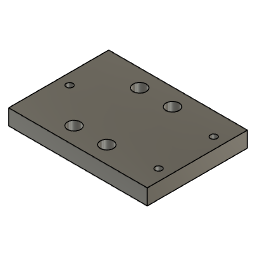
Fixation_camera v4 (Autodesk Fusion 360 design; units mm, degrees)
Autodesk Fusion 360 part; units mm, degrees
sketch "Esquisse1" plane through (0, 0, 0) normal (0, 0, 1) x (1, 0, 0)
  circle A0 centre (-12.5, 4.445) radius 2.5
  circle A1 centre (-12.5, -8.055) radius 2.5
  circle A2 centre (12.5, 4.445) radius 2.5
  circle A3 centre (-10.5, 22.15) radius 1.25
  line L0 (-14.5, -24.35) -> (-14.5, 24.35) construction
  line L1 (19.05, -25.4) -> (19.05, 25.4)
  line L2 (-19.05, -25.4) -> (-19.05, 25.4)
  circle A4 centre (12.5, -8.055) radius 2.5
  line L3 (-19.05, -25.4) -> (19.05, -25.4)
  line L4 (-19.05, 25.4) -> (-19.05, -25.4)
  line L5 (14.5, 24.35) -> (14.5, -24.35) construction
  line L6 (19.05, 25.4) -> (19.05, -25.4)
  line L7 (19.05, 25.4) -> (-19.05, 25.4)
  circle A5 centre (-12.5, -8.055) radius 2.5
  line L8 (14.5, -24.35) -> (-14.5, -24.35) construction
  circle A6 centre (10.5, 22.15) radius 1.25
  line L9 (-19.05, 25.4) -> (19.05, 25.4)
  circle A7 centre (12.5, 4.445) radius 2.5
  line L10 (19.05, -25.4) -> (-19.05, -25.4)
  circle A8 centre (0, -22.25) radius 1.25
  circle A9 centre (-12.5, 4.445) radius 2.5
  line L11 (-14.5, 24.35) -> (14.5, 24.35) construction
  circle A10 centre (12.5, -8.055) radius 2.5
  dimension "d1" = 38.1
  dimension "d2" = 50.8
  dimension "d5" = 29
  dimension "d7" = 48.7
  dimension "d9" = 2.2
  dimension "d10" = 2.2
  dimension "d11" = 14.5
  dimension "d12" = 2.5
  dimension "d13" = 2.5
  dimension "d14" = 2.5
  dimension "d15" = 21
  dimension "d16" = 44.4
  dimension "d17" = 5
  dimension "d18" = 5
  dimension "d19" = 5
  dimension "d20" = 5
  constraint horizontal L9
  constraint vertical L6
  constraint horizontal L10
  constraint vertical L2
  constraint horizontal L11
  constraint vertical L5
  constraint horizontal L8
  constraint vertical L0
  constraint concentric A0 A9
  constraint concentric A2 A7
  constraint concentric A1 A5
  constraint concentric A4 A10
  measures "d1" distance of L2 L6
  measures "d2" distance of L9 L10
  measures "d5" distance of L0 L5
  measures "d7" distance of L8 L11
  measures "d9" distance of A3.centre L11
  measures "d10" distance of A6.centre L11
  measures "d11" distance of A8.centre L0
  measures "d12" diameter of A3
  measures "d13" diameter of A6
  measures "d14" diameter of A8
  measures "d15" distance of A6.centre A3.centre
  measures "d16" vertical distance of A3.centre A8.centre
  measures "d17" diameter of A9
  measures "d18" diameter of A7
  measures "d19" diameter of A5
  measures "d20" diameter of A10
extrude "Extrusion1" add sketch "Esquisse1" along normal blind 5.95
extrude "Extrusion2" add 1 faces at (-6.35, -25.4, 3.9667) along direction (0, -1, 0) blind 1
extrude "Extrusion3" add 1 faces at (6.35, 25.4, 3.9667) along direction (0, 1, 0) blind 1
move_body "Déplacer1" bodies 1 to x (0, -1, 0) y (1, 0, 0) z (0, 0, 1) at (0, 0, 0)
